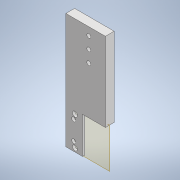
# Autodesk Inventor part: endcap insert
Saved by Autodesk Inventor 2022 (Build 260153000, 153)
## iProperties
Created: 2021-11-30
Part Number: endcap insert
Material: Generic
Document SubType Name: Modeling
Designer: efred
Density: 1 g/cm^3
Appearance: Default
Author: efred
Autodesk Inventor part; units mm, degrees
ref_plane "YZ Plane" through (0, 0, 0) normal (1, 0, 0) x (0, 1, 0)
ref_plane "XZ Plane" through (0, 0, 0) normal (0, 1, 0) x (-1, 0, 0)
ref_plane "XY Plane" through (0, 0, 0) normal (0, 0, 1) x (1, 0, 0)
ref_plane "Work Plane1" through (0, 0, 0) normal (0, 0, 1) x (1, 0, 0)
sketch "Sketch1" plane through (0, 0, 0) normal (0, 0, 1) x (1, 0, 0)
  circle A0 centre (-13.5, -18.5) radius 3.15 projected
  circle A1 centre (-13.5, 18.5) radius 3.15 projected
  line L0 (-25, -23) -> (25, -23) construction
  line L1 (25, -23) -> (25, 23) projected
  line L2 (25, 23) -> (-25, 23) construction
  line L3 (-25, 23) -> (-25, -23) construction
  circle A2 centre (-15, 12) radius 2.65 projected
  circle A3 centre (-15, -12) radius 2.65 projected
  circle A4 centre (12, 0) radius 4.15 projected
  line L4 (-25, -11.95) -> (-20, -11.95) construction
  line L5 (-20, -11.95) -> (-20, -7.95) construction
  line L6 (-20, -7.95) -> (-25, -7.95) construction
  line L7 (-25, 7.95) -> (-25, -7.95) construction
  line L8 (-25, 7.95) -> (-20, 7.95) construction
  line L9 (-20, 7.95) -> (-20, 11.95) construction
  line L10 (-20, 11.95) -> (-25, 11.95) construction
  line L11 (-25, 19.95) -> (-25, 11.95) construction
  line L12 (-25, 19.95) -> (-4, 19.95) construction
  line L13 (-4, 11.95) -> (-4, 19.95) construction
  line L14 (-4, 11.95) -> (-9, 11.95) construction
  line L15 (-9, 11.95) -> (-9, 7.95) construction
  line L16 (-9, 7.95) -> (-4, 7.95) construction
  line L17 (-4, -7.95) -> (-4, 7.95) construction
  line L18 (-4, -7.95) -> (-9, -7.95) construction
  line L19 (-9, -7.95) -> (-9, -11.95) construction
  line L20 (-9, -11.95) -> (-4, -11.95) construction
  line L21 (-4, -19.95) -> (-4, -11.95) construction
  line L22 (-4, -19.95) -> (-25, -19.95) construction
  line L23 (-25, -11.95) -> (-25, -19.95) construction
  line L24 (-4, -23.1) -> (-25, -23.1)
  line L25 (-25, -23.1) -> (-25, 23.1)
  line L26 (-25, 23.1) -> (-4, 23.1)
  line L27 (-4, 23.1) -> (-4, -23.1)
  point P0 (0, 0)
  dimension "d3" = 0.1
  dimension "d4" = 0.1
  constraints: 8 end point, 2 collinear, 2 parallel, 1 horizontal, 1 perpendicular
  measures "d3" distance between parallel lines of L0 L24
  measures "d4" distance between parallel lines of L2 L26
extrude "Extrusion1" add sketch "Sketch1" along normal blind 3 contours L24 L25 L26 L27
sketch "Sketch3" plane through (-25, 23.1, 0) normal (0, 1, 0) x (1, 0, 0)
  line L0 (50, 8.1) -> (0, 8.1) construction
  line L1 (0, 8.1) -> (0, 0.1) construction
  line L2 (50, 0.1) -> (0, 0.1) construction
  line L3 (50, 8.1) -> (50, 0.1) construction
  line L4 (21, 0) -> (0, 0) construction
  line L5 (0, 0) -> (0, -3) construction
  line L6 (21, -3) -> (0, -3) construction
  line L7 (21, 0) -> (21, -3) construction
  line L8 (21, -3) -> (0, -3) projected
  line L9 (0, -3) -> (50, -3)
  line L10 (50, -3) -> (50, 8.1)
  line L11 (50, 8.1) -> (0, 8.1)
  line L12 (0, 8.1) -> (0, -3)
  point P0 (25, 0)
  constraints: 8 end point, 2 parallel, 1 horizontal, 1 perpendicular
extrude "Extrusion2" add sketch "Sketch3" along normal blind 100
sketch "Sketch5" plane through (-25, -23.1, 0) normal (-1, 0, 0) x (0, 0, 1)
  circle A0 centre (-2.55, 126.2) radius 2.65 construction
  circle A1 centre (-2.55, 106.2) radius 2.65 construction
  circle A2 centre (-2.55, 86.2) radius 2.65 construction
  circle A3 centre (-2.55, 66.2) radius 2.65 construction
  circle A4 centre (-2.55, 126.2) radius 2.5
  line L0 (-2.55, 126.2) -> (-2.55, 106.2) construction
  circle A5 centre (-2.55, 106.2) radius 2.5
  circle A6 centre (-2.55, 86.2) radius 2.5
  circle A7 centre (-2.55, 66.2) radius 2.5
  point P0 (0, 23.1)
  dimension "d17" = 5
  dimension "d20" = 20
  constraints: 4 centre point, 2 end point, 2 vertical, 1 coincident, 6 other
  measures "d17" diameter of A4
  measures "d20" distance of L0.start A5.centre
extrude "Extrusion4" cut sketch "Sketch5" against normal blind 25
sketch "Sketch6" plane through (0, 0, 3) normal (0, 0, 1) x (1, 0, 0)
  circle A0 centre (4, 83.1) radius 2.65 construction
  circle A1 centre (4, 98.1) radius 2.65 construction
  circle A2 centre (4, 113.1) radius 2.65 construction
  circle A3 centre (4, 83.1) radius 2.5
  circle A4 centre (4, 98.1) radius 2.5
  circle A5 centre (4, 113.1) radius 2.5
  point P0 (0, 0)
  dimension "d27" = 5
  dimension "d28" = 5
  dimension "d29" = 5
  constraints: 3 centre point, 3 coincident
  measures "d27" diameter of A5
  measures "d28" diameter of A4
  measures "d29" diameter of A3
extrude "Extrusion5" cut sketch "Sketch6" against normal through all
equation "\"d4\" = d3"
body "Solid1"
